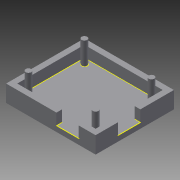
# Autodesk Inventor part: Casing Bottom
Saved by Autodesk Inventor 2014 SP1 (Build 180222100, 222)
## iProperties
Created: 2013-10-01
Part Number: Casing Bottom
Material: Generic
Document SubType Name: Modeling
Designer: Anthony
Density: 1 g/cm^3
Appearance: Default
Author: Anthony
Autodesk Inventor part; units mm, degrees
ref_plane "YZ Plane" through (0, 0, 0) normal (1, 0, 0) x (0, 1, 0)
ref_plane "XZ Plane" through (0, 0, 0) normal (0, 1, 0) x (-1, 0, 0)
ref_plane "XY Plane" through (0, 0, 0) normal (0, 0, 1) x (1, 0, 0)
sketch "Sketch1" plane through (0, 0, 0) normal (0, 1, 0) x (-1, 0, 0)
  line L0 (0, 0) -> (-50.8, 0)
  line L1 (-50.8, 0) -> (-50.8, 44.45)
  line L2 (-50.8, 44.45) -> (0, 44.45)
  line L3 (0, 44.45) -> (0, 0)
  dimension "d0" = 44.45
  dimension "d1" = 50.8
  constraints: 8 end point, 2 parallel, 1 horizontal, 1 perpendicular
  measures "d0" distance of L0.end L1.end
  measures "d1" distance of L1.end L2.end
extrude "Extrusion1" add sketch "Sketch1" along normal blind 3.175
sketch "Sketch2" plane through (0, 3.175, 0) normal (0, 1, 0) x (1, 0, 0)
  line L0 (50.8, 0) -> (0, 0) projected
  line L1 (0, 0) -> (0, -44.45) projected
  line L2 (0, -44.45) -> (50.8, -44.45) projected
  line L3 (50.8, -44.45) -> (50.8, 0) projected
  line L4 (3.175, -3.175) -> (47.625, -3.175)
  line L5 (47.625, -3.175) -> (47.625, -41.275)
  line L6 (47.625, -41.275) -> (3.175, -41.275)
  line L7 (3.175, -41.275) -> (3.175, -3.175)
  dimension "d4" = 3.175
  dimension "d5" = 3.175
  dimension "d6" = 3.175
  dimension "d7" = 3.175
  constraints: 8 end point, 2 parallel, 1 horizontal, 1 perpendicular
  measures "d4" distance between parallel lines of L1 L7
  measures "d5" distance between parallel lines of L0 L4
  measures "d6" distance between parallel lines of L2 L6
  measures "d7" distance between parallel lines of L3 L5
extrude "Extrusion2" add sketch "Sketch2" along normal blind 6.35
sketch "Sketch3" plane through (0, 3.175, 0) normal (0, 1, 0) x (1, 0, 0)
  line L0 (47.625, -41.275) -> (47.625, -3.175) projected
  line L1 (47.625, -3.175) -> (3.175, -3.175) projected
  line L2 (3.175, -3.175) -> (3.175, -41.275) projected
  line L3 (3.175, -41.275) -> (47.625, -41.275) projected
  circle A0 centre (6.35, -38.1) radius 1.5875
  circle A1 centre (6.35, -6.35) radius 1.5875
  circle A2 centre (44.45, -6.35) radius 1.5875
  circle A3 centre (44.45, -38.1) radius 1.5875
  point P0 (0, 0)
  dimension "d10" = 3.175
  dimension "d11" = 3.175
  dimension "d12" = 3.175
  dimension "d13" = 3.175
  dimension "d14" = 3.175
  dimension "d15" = 3.175
  dimension "d16" = 3.175
  dimension "d17" = 3.175
  dimension "d18" = 3.175
  dimension "d19" = 3.175
  dimension "d20" = 3.175
  dimension "d21" = 3.175
  constraints: 4 centre point
  measures "d10" diameter of A1
  measures "d11" diameter of A0
  measures "d12" diameter of A3
  measures "d13" diameter of A2
  measures "d14" distance from line of L3 A0.centre
  measures "d15" distance from line of L2 A0.centre
  measures "d16" distance from line of L2 A1.centre
  measures "d17" distance from line of L1 A1.centre
  measures "d18" distance from line of L1 A2.centre
  measures "d19" distance from line of L0 A2.centre
  measures "d20" distance from line of L0 A3.centre
  measures "d21" distance from line of L3 A3.centre
extrude "Extrusion3" add sketch "Sketch3" along normal blind 12.7 contours A0 | A1 | A2 | A3
sketch "Sketch4" plane through (0, 0, 44.45) normal (0, 0, 1) x (1, 0, 0)
  line L0 (0, 9.525) -> (50.8, 9.525) projected
  line L1 (0, 0) -> (0, 9.525) projected
  line L2 (28.575, 9.525) -> (41.275, 9.525)
  line L3 (41.275, 9.525) -> (41.275, 3.175)
  line L4 (41.275, 3.175) -> (28.575, 3.175)
  line L5 (28.575, 3.175) -> (28.575, 9.525)
  dimension "d24" = 6.35
  dimension "d25" = 28.575
  dimension "d27" = 41.275
  constraints: 8 end point, 2 parallel, 1 horizontal, 1 perpendicular, 1 point on line
  measures "d24" distance of L4.end L2.start
  measures "d25" distance from line of L1.start L5
  measures "d27" distance between parallel lines of L1 L3
extrude "Extrusion4" cut sketch "Sketch4" against normal blind 3.175
sketch "Sketch5" plane through (50.8, 0, 44.45) normal (1, 0, 0) x (0, 0, -1)
  line L0 (0, 9.525) -> (44.45, 9.525) projected
  line L1 (0, 0) -> (0, 9.525) projected
  line L2 (12.7, 9.525) -> (25.4, 9.525)
  line L3 (25.4, 9.525) -> (25.4, 3.175)
  line L4 (25.4, 3.175) -> (12.7, 3.175)
  line L5 (12.7, 3.175) -> (12.7, 9.525)
  dimension "d30" = 12.7
  dimension "d31" = 25.4
  dimension "d32" = 6.35
  constraints: 8 end point, 2 parallel, 1 horizontal, 1 perpendicular, 1 point on line
  measures "d30" distance between parallel lines of L1 L5
  measures "d31" distance between parallel lines of L3 L1
  measures "d32" distance between parallel lines of L0 L4
extrude "Extrusion5" cut sketch "Sketch5" against normal blind 3.175
sketch "Sketch6" plane through (0, 3.175, 0) normal (0, 1, 0) x (1, 0, 0)
  circle A0 centre (44.45, -6.35) radius 1.5875 projected
  circle A1 centre (6.35, -38.1) radius 1.5875 projected
  circle A2 centre (6.35, -6.35) radius 1.5875 projected
  circle A3 centre (44.45, -38.1) radius 1.5875 projected
  line L0 (47.625, -41.275) -> (47.625, -31.75) projected
  line L1 (50.8, -31.75) -> (47.625, -31.75) projected
  line L2 (50.8, -19.05) -> (50.8, -31.75) projected
  line L3 (50.8, -19.05) -> (47.625, -19.05) projected
  line L4 (47.625, -19.05) -> (47.625, -3.175) projected
  line L5 (47.625, -3.175) -> (3.175, -3.175) projected
  line L6 (3.175, -3.175) -> (3.175, -41.275) projected
  line L7 (3.175, -41.275) -> (28.575, -41.275) projected
  line L8 (28.575, -44.45) -> (28.575, -41.275) projected
  line L9 (41.275, -44.45) -> (28.575, -44.45) projected
  line L10 (41.275, -44.45) -> (41.275, -41.275) projected
  line L11 (41.275, -41.275) -> (47.625, -41.275) projected
  point P0 (0, 0)
body "Solid1"
